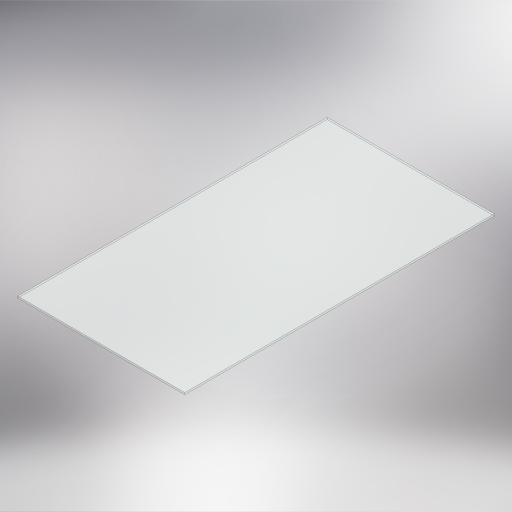
# Autodesk Inventor part: Glass Slide Spacer V1
Saved by Autodesk Inventor 2024 (Build 280153000, 153)
## iProperties
Created: 2024-03-20
Part Number: Glass Slide Spacer V1
Material: Glass
Document SubType Name: Modeling
Designer: cfang
Density: 2.18 g/cm^3
Appearance: Clear
Author: cfang
Autodesk Inventor part; units mm, degrees
ref_plane "YZ Plane" through (0, 0, 0) normal (1, 0, 0) x (0, 1, 0)
ref_plane "XZ Plane" through (0, 0, 0) normal (0, 1, 0) x (-1, 0, 0)
ref_plane "XY Plane" through (0, 0, 0) normal (0, 0, 1) x (1, 0, 0)
sketch "Sketch1" plane through (0, 0, 0) normal (0, 1, 0) x (-1, 0, 0)
  line L0 (-11.5, -21.3) -> (11.5, -21.3)
  line L1 (11.5, -21.3) -> (11.5, 21.3)
  line L2 (11.5, 21.3) -> (-11.5, 21.3)
  line L3 (-11.5, 21.3) -> (-11.5, -21.3)
  line L4 (-11.5, -21.3) -> (11.5, 21.3) construction
  line L5 (11.5, -21.3) -> (-11.5, 21.3) construction
  point P0 (0, 0)
  dimension "d0" = 42.6
  dimension "d1" = 23
  constraints: 12 end point, 2 midpoint, 2 parallel, 1 horizontal, 1 perpendicular
  measures "d0" distance of L0.end L1.end
  measures "d1" distance of L1.end L2.end
extrude "Extrusion1" add sketch "Sketch1" along normal blind 0.25
body "Solid1"
